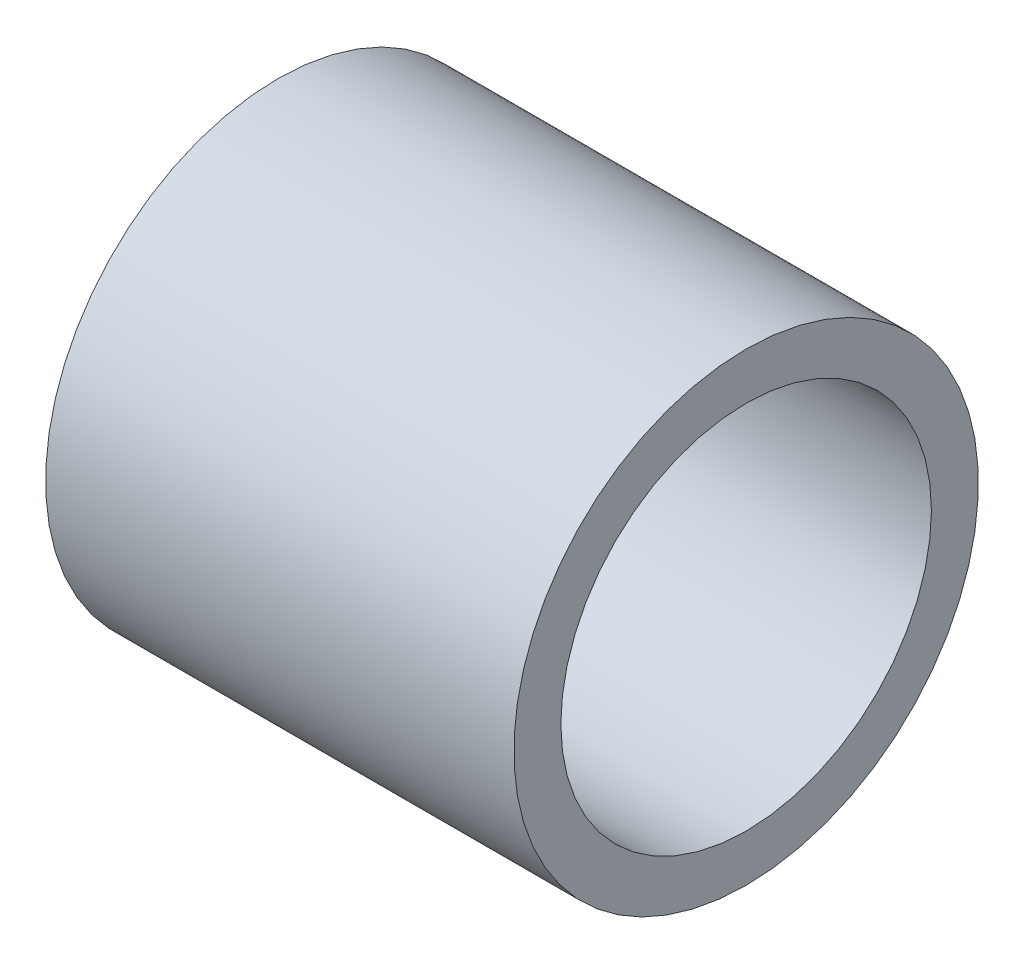
# Autodesk Inventor part: TruckBushing
Saved by Autodesk Inventor 2015 SP1 (Build 190203100, 203)
## iProperties
Created: 2015-06-30
Part Number: TruckBushing
Material: ABS Plastic
Document SubType Name: Modeling
Designer: YOUR_NAME_HERE
Density: 1.06 g/cm^3
Appearance: Smooth - Yellow
Author: YOUR_NAME_HERE
Autodesk Inventor part; units mm, degrees
ref_plane "YZ Plane" through (0, 0, 0) normal (1, 0, 0) x (0, 1, 0)
ref_plane "XZ Plane" through (0, 0, 0) normal (0, 1, 0) x (-1, 0, 0)
ref_plane "XY Plane" through (0, 0, 0) normal (0, 0, 1) x (1, 0, 0)
sketch "Sketch1" plane through (0, 0, 0) normal (1, 0, 0) x (0, 1, 0)
  circle A0 centre (0, 0) radius 7.5381
  circle A1 centre (0, 0) radius 9.4488
  dimension "d1" = 18.8976
  dimension "d2" = 15.0762
  constraints: 2 centre point, 1 coincident
  measures "d1" diameter of A1
  measures "d2" diameter of A0
extrude "Extrusion1" add sketch "Sketch1" along normal blind 19.05
body "Solid1"
